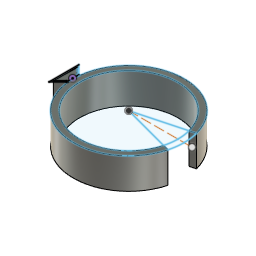
cup_ring_v2 (Autodesk Fusion 360 design; units mm, degrees)
Autodesk Fusion 360 part; units mm, degrees
sketch "Sketch1" plane through (0, 0, 0) normal (0, 0, 1) x (1, 0, 0)
  line L0 (0, 0) -> (0, -5)
  line L1 (0, 0) -> (0, 5)
  line L2 (0, 5) -> (-7.0711, 12.0711)
  line L3 (0, -5) -> (-7.0711, -12.0711)
  line L4 (-7.0711, -12.0711) -> (-7.0711, 12.0711)
  circle A0 centre (45.5796, 0.0284) radius 40
  circle A1 centre (45.5796, 0.0284) radius 45
  line L5 (0, 5) -> (0.855, 5)
  line L6 (0, -5) -> (0.8614, -5)
  line L7 (-0.7071, -4.2929) -> (-6.0711, -9.6569)
  line L8 (-6.0711, -9.6569) -> (-6.0711, 9.6569)
  line L9 (-0.7071, 4.2929) -> (-6.0711, 9.6569)
  line L10 (-0.7071, 4.2929) -> (0.7821, 4.2929)
  line L11 (-0.7071, -4.2929) -> (0.7875, -4.2929)
  line L12 (45.5796, 0.0284) -> (97, 0.0284) construction
  line L13 (45.5796, 0.0284) -> (89.0462, -11.6185)
  line L14 (45.5796, 0.0284) -> (89.0462, 11.6752)
  dimension "d1" = 5
  dimension "d2" = 10
  dimension "d3" = 10
  dimension "d4" = 80
  dimension "d5" = 5
  dimension "d6" = 1
  dimension "d11" = 15
  dimension "d12" = 15
  constraint coincident L0.start L1.start
  constraint vertical L0
  constraint parallel L0 L1
  constraint perpendicular L2 L3
  constraint vertical L4
  constraint coincident A1 L5.end
  constraint perpendicular L1 L5
  constraint coincident A1 L6.end
  constraint perpendicular L0 L6
  constraint coincident A1 L10.end
  constraint perpendicular L1 L10
  constraint coincident A1 L11.end
  constraint perpendicular L0 L11
  constraint coincident A0.centre A1.centre
  constraint horizontal L12
  constraint coincident A1 L13.end
  constraint coincident A1 L14.end
  measures "d1" distance of L0.start L0.end
  measures "d2" distance of L1.end L2.end
  measures "d3" distance of L0.end L3.end
  measures "d4" diameter of A0
  measures "d11" angle of L12 L13
  measures "d12" angle of L12 L14
extrude "Extrude3" add sketch "Sketch1" against normal blind 15 contours A0 A1 L13 L14 picked at (87.9713, -8.774) makes body 1
extrude "Extrude1" add sketch "Sketch1" against normal blind 25 separate body contours L0 L1 A1 L10 L11 | L0 L1 L7 L8 L9 L10 L11 makes body 2
combine "Combine1" operation cut target body 2 tool bodies 1
extrude "Extrude4" add sketch "Sketch1" against normal blind 25 contours A0 A1 L13 L14 picked at (3.1611, -8.3994) bodies 2
